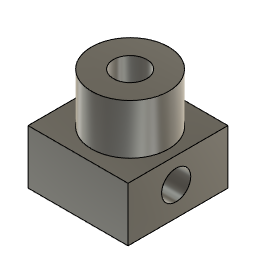
Baseplate Holder (Autodesk Fusion 360 design; units mm, degrees)
Autodesk Fusion 360 part; units mm, degrees
box "BoxPrimitive1" add length 38.0931 width 38.1 height 20.6375 placed x (0, -1, 0) y (1, 0, 0) z (0, 0, 1) at (0, 0, 0)
cylinder "CylinderPrimitive1" add diameter 29.3624 height 19.05 placed x (1, 0, 0) y (0, 1, 0) z (0, 0, 1) at (19.8488, -19.0466, 20.6375)
hole "Hole1" at (19.8488, -19.0466, 39.6875) direction (0, 0, -1) diameter 12.7 depth 35.2044 tip angle 180
hole "Hole2" at (38.1, -19.7481, 10.9094) direction (-1, 0, 0) diameter 11.1201 depth 18.1864 tip angle 180
